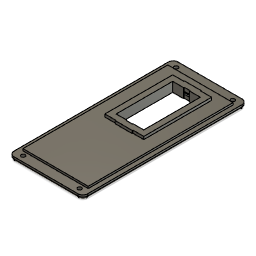
TampaBat12V (Autodesk Fusion 360 design; units mm, degrees)
Autodesk Fusion 360 part; units mm, degrees
sketch "Esboço1" plane through (0, 0, 0) normal (0, 1, 0) x (1, 0, 0)
  line L0 (0, -5) -> (0, -164)
  arc A0 (71, -169) -> (76, -164) centre (71, -164) ccw
  circle A1 centre (67.1121, -163.3) radius 2
  arc A2 (76, -5) -> (71, 0) centre (71, -5) ccw
  line L1 (4, -9.5) -> (72, -9.5)
  circle A3 centre (67.1121, -5.7) radius 2
  arc A4 (5, 0) -> (0, -5) centre (5, -5) ccw
  line L2 (72, -9.5) -> (72, -159.5)
  circle A5 centre (8.8879, -163.3) radius 2
  line L3 (72, -159.5) -> (4, -159.5)
  arc A6 (0, -164) -> (5, -169) centre (5, -164) ccw
  line L4 (76, -164) -> (76, -5)
  circle A7 centre (8.8879, -5.7) radius 2
  line L5 (71, 0) -> (5, 0)
  line L6 (4, -159.5) -> (4, -9.5)
  line L7 (5, -169) -> (71, -169)
extrude "Extrusão1" add sketch "Esboço1" along normal blind 5 contours L0 A0 A2 A4 A6 L4 L5 L7 | L1 L2 L3 L6
sketch "Esboço3" plane through (0, 5, 0) normal (0, 1, 0) x (-1, 0, 0)
  circle A0 centre (-8.8879, 163.3) radius 2
  circle A1 centre (-67.1121, 5.7) radius 2
  circle A2 centre (-67.1121, 163.3) radius 2
  circle A3 centre (-8.8879, 5.7) radius 2
  line L0 (-5, 169) -> (-71, 169)
  arc A4 (-71, 169) -> (-76, 164) centre (-71, 164) ccw
  line L1 (-76, 164) -> (-76, 5)
  arc A5 (-76, 5) -> (-71, 0) centre (-71, 5) ccw
  line L2 (-71, 0) -> (-5, 0)
  arc A6 (-5, 0) -> (0, 5) centre (-5, 5) ccw
  line L3 (0, 5) -> (0, 164)
  arc A7 (0, 164) -> (-5, 169) centre (-5, 164) ccw
  line L4 (-76, 164) -> (-76, 5)
  arc A8 (-5, 0) -> (0, 5) centre (-5, 5) ccw
  circle A9 centre (-8.8879, 5.7) radius 2
  arc A10 (0, 164) -> (-5, 169) centre (-5, 164) ccw
  line L5 (-72, 159.5) -> (-4, 159.5)
  circle A11 centre (-8.8879, 163.3) radius 2
  arc A12 (-71, 169) -> (-76, 164) centre (-71, 164) ccw
  line L6 (-4, 159.5) -> (-4, 9.5)
  circle A13 centre (-67.1121, 5.7) radius 2
  line L7 (-4, 9.5) -> (-72, 9.5)
  arc A14 (-76, 5) -> (-71, 0) centre (-71, 5) ccw
  line L8 (0, 5) -> (0, 164)
  circle A15 centre (-67.1121, 163.3) radius 2
  line L9 (-5, 169) -> (-71, 169)
  line L10 (-72, 9.5) -> (-72, 159.5)
  line L11 (-71, 0) -> (-5, 0)
  line L12 (-71.6, 159.1) -> (-4.4, 159.1)
  line L13 (-4.4, 159.1) -> (-4.4, 9.9)
  line L14 (-4.4, 9.9) -> (-71.6, 9.9)
  line L15 (-71.6, 9.9) -> (-71.6, 159.1)
  point P0 (-76, 169)
  dimension "d3" = 0.4
extrude "Extrusão2" add sketch "Esboço3" along normal blind 2 contours L12 L13 L14 L15
sketch "Esboço4" plane through (0, 7, 0) normal (0, 1, 0) x (-1, 0, 0)
  line L0 (-71.6, 9.9) -> (-4.4, 9.9)
  line L1 (-4.4, 9.9) -> (-4.4, 159.1)
  line L2 (-4.4, 159.1) -> (-71.6, 159.1)
  line L3 (-71.6, 159.1) -> (-71.6, 9.9)
  line L4 (-52.7, 24.8) -> (-52.7, 83)
  line L5 (-35.5, 24.2) -> (-41.5, 24.2)
  line L6 (-24.3, 24.8) -> (-35.5, 24.8)
  line L7 (-41.5, 24.2) -> (-41.5, 24.8)
  line L8 (-24.3, 83) -> (-24.3, 24.8)
  line L9 (-52.7, 83) -> (-41.5, 83)
  line L10 (-41.5, 24.8) -> (-52.7, 24.8)
  line L11 (-41.5, 83.6) -> (-35.5, 83.6)
  line L12 (-35.5, 83.6) -> (-35.5, 83)
  line L13 (-35.5, 83) -> (-24.3, 83)
  line L14 (-41.5, 83) -> (-41.5, 83.6)
  line L15 (-35.5, 24.8) -> (-35.5, 24.2)
  line L16 (-29.6883, 89.4117) -> (-29.6883, 88.8117)
  line L17 (-29.6883, 88.8117) -> (-18.4883, 88.8117)
  line L18 (-18.4883, 88.8117) -> (-18.4883, 18.9883)
  line L19 (-18.4883, 18.9883) -> (-29.6883, 18.9883)
  line L20 (-29.6883, 18.9883) -> (-29.6883, 18.3883)
  line L21 (-29.6883, 18.3883) -> (-47.3117, 18.3883)
  line L22 (-47.3117, 18.3883) -> (-47.3117, 18.9883)
  line L23 (-47.3117, 18.9883) -> (-58.5117, 18.9883)
  line L24 (-58.5117, 18.9883) -> (-58.5117, 88.8117)
  line L25 (-58.5117, 88.8117) -> (-47.3117, 88.8117)
  line L26 (-47.3117, 88.8117) -> (-47.3117, 89.4117)
  line L27 (-47.3117, 89.4117) -> (-29.6883, 89.4117)
  dimension "d6" = -5.8117
extrude "Extrusão3" add sketch "Esboço4" along normal blind 2.8 contours L16 L17 L18 L19 L20 L21 L22 L23 L24 L25 L26 L27
extrude "Extrusão4" cut 1 faces at (48.9667, 7, 44.2) along direction (0, -1, 0) blind 14
sketch "Esboço5" plane through (0, 0, 83.6) normal (0, 0, -1) x (-1, 0, 0)
  line L0 (-35.5, 0) -> (-35.5, 9.8)
  line L1 (-35.5, 9.8) -> (-41.5, 9.8)
  line L2 (-41.5, 9.8) -> (-41.5, 0)
  line L3 (-41.5, 0) -> (-35.5, 0)
  line L4 (-35.5, 4.9) -> (-36, 4.9)
  line L5 (-36, 4.9) -> (-41.5, 4.9)
  line L6 (-35.5, 5) -> (-36, 5)
  line L7 (-36, 5) -> (-41.5, 5)
  line L8 (-35.5, 4.8) -> (-36, 4.8)
  line L9 (-36, 4.8) -> (-41.5, 4.8)
  dimension "d11" = 0.1
  dimension "d12" = -0.1
  constraint midpoint L0 L4.start
  constraint perpendicular L0 L4
  constraint midpoint L2 L5.end
  constraint perpendicular L2 L5
extrude "Extrusão5" cut sketch "Esboço5" against normal blind 0.3 contours L0 L2 L4 L5 L8 L9 | L0 L2 L4 L5 L6 L7
chamfer "Chanfro1" distance 1.2 distance2 0.3 1 edges at (38.5, 5, 83.6) measured on face at (39.5, 8.2, 83.6)
chamfer "Chanfro2" distance 1.2 distance2 0.3 1 edges at (38.5, 4.8, 83.6) measured on face at (39.5, 3.2, 83.6)
sketch "Esboço6" plane through (0, 0, 24.2) normal (0, 0, 1) x (1, 0, 0)
  line L0 (41.5, 0) -> (41.5, 9.8)
  line L1 (41.5, 9.8) -> (35.5, 9.8)
  line L2 (35.5, 9.8) -> (35.5, 0)
  line L3 (35.5, 0) -> (41.5, 0)
  line L4 (35.5, 4.9) -> (41.5, 4.9)
  line L5 (35.5, 4.8) -> (41.5, 4.8)
  line L6 (35.5, 5) -> (41.5, 5)
  dimension "d19" = 0.1
  dimension "d20" = -0.1
  constraint midpoint L2 L4.start
  constraint midpoint L0 L4.end
extrude "Extrusão6" cut sketch "Esboço6" against normal blind 0.3 contours L0 L2 L4 L5 | L0 L2 L4 L6
chamfer "Chanfro3" distance 1.2 distance2 0.3 1 edges at (38.5, 5, 24.2) measured on face at (37.5, 8.2, 24.2)
chamfer "Chanfro4" distance 1.2 distance2 0.3 1 edges at (38.5, 4.8, 24.2) measured on face at (37.5, 3.2, 24.2)
fillet "Arredondamento1" radius 3 8 edges at (0, 0, 84.5) (1.4645, 0, 167.5355) (38, 0, 169) (74.5355, 0, 167.5355) (76, 0, 84.5) (74.5355, 0, 1.4645) (38, 0, 0) (1.4645, 0, 1.4645)
